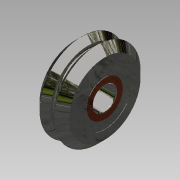
# Autodesk Inventor part: W3X
Saved by Autodesk Inventor 2020.1 (Build 241239000, 239)
## iProperties
Created: 2019-11-27
Part Number: W3X
Material: Generic
Catalog Web Link: https://www.bwc.com/dualvee.html
Vendor: BWC
Document SubType Name: Modeling
Designer: Autodesk Inc.
Manufacturer: BWC
Mass: 130.2 g
Surface Area: 59.8551 cm^2
Volume: 19.8505 cm^3
Density: 1 g/cm^3
Appearance: PSOLRGB-175-175-175
Category: FIRSTChoice
Company: Autodesk Inc.
PSOL_IDENT_0: {$CADENAS_DATA\23d-libs\bwc\dual_vee\wheels\original_dualvee_wheels.prj},163 {VTYP=3D},{NB=W3X},{LIN
PSOL_IDENT_1: A=W3X},{NN=Original DualVee Wheels},{DATE=01.07.2019 05:07:11},{GEOMDATE=12.02.2019 13:07:27},{VERSI
PSOL_IDENT_2: ON=},{LINEID=40},{WBVAR=},{WBNUMERIC=}  {NB=W3X},{LINA=W3X},{KT=DUMMY},{PN=W3X},{WS=WX Steel Seal/Sh
PSOL_IDENT_3: ield},{WSPN=X},{WSALG= 'X','WX Seal/Shield Steel', 'SSX','WSSX Seal/Shield Stainless Steel','SS227',
PSOL_IDENT_4: 'WSS227 Shield Stainless Steel Krytox GPL227 Lubricant','SS300', 'WSS300 Stainless Steel Isoflex PD
PSOL_IDENT_5: L 300 (grease, no shields or seals)','DW3SSX', 'Washdown Sealed Wheels' },{SIZE=3},{D=1.803},{W=0.62
PSOL_IDENT_6: 5},{B=0.4724},{VRI=0.750},{VRO=1.063},{WEIGHT=130.2},{C=0.755},{R=0.039},{R1=0.024},{E=0.010},{RLN=5
PSOL_IDENT_7: 900},{RLLBF=1326},{ALN=1701},{ALLBF=382},{ORMAT=52100 Steel},{IRMAT=52100 Steel},{BMAT=52100 Steel},
PSOL_IDENT_8: {RMAT=Nylon 6,6},{SHMAT=304 Stainless steel},{SMAT=NBR+304 Stainless steel},{GREASE=Kluberplex BEM 3
PSOL_IDENT_9: 4-132},{CFGFILTER=PN,WS,SIZE,D,W,B,VRI,VRO,WEIGHT,RLN,RLLBF,ALN,ALLBF,ORMAT,IRMAT,BMAT,RMAT,SHMAT,SM
PSOL_IDENT_10: AT,GREASE},{CATEGALG=Original Guide Wheel, Size 3, Carbon Steel, Sealed/Shielded},{FEATALG=<li style=
PSOL_IDENT_11: \" margin-top:0px; margin-bottom:0px; margin-left:0px; margin-right:0px; -qt-block-indent:0; text-in
PSOL_IDENT_12: dent:0px;\"><span style=\" font-size:11pt; font-weight:600;\">General purpose AISI 52100 carbon stee
PSOL_IDENT_13: l</span></li><li style=\" font-size:11pt; font-weight:600;\" style=\" margin-top:0px; margin-bottom:
PSOL_IDENT_14: 0px; margin-left:0px; margin-right:0px; -qt-block-indent:0; text-indent:0px;\">Double row angular co
PSOL_IDENT_15: ntact ball bearing</li><li style=\" font-size:11pt; font-weight:600;\" style=\" margin-top:0px; marg
PSOL_IDENT_16: in-bottom:0px; margin-left:0px; margin-right:0px; -qt-block-indent:0; text-indent:0px;\">Precision g
PSOL_IDENT_17: round 90° vee inside or outside running surfaces</li><li style=\" font-size:11pt; font-weight:600;\"
PSOL_IDENT_18: style=\" margin-top:0px; margin-bottom:0px; margin-left:0px; margin-right:0px; -qt-block-indent:0;
PSOL_IDENT_19: text-indent:0px;\">Hardened for heavy loads and durability</li><li style=\" font-size:11pt; font-wei
PSOL_IDENT_20: ght:600;\" style=\" margin-top:0px; margin-bottom:0px; margin-left:0px; margin-right:0px; -qt-block-
PSOL_IDENT_21: indent:0; text-indent:0px;\">Seal/Shield combination to protect against contamination</li>},{DESCRAL
PSOL_IDENT_22: G=<span style=\" font-size:11pt; font-weight:600;\">DualVee WX series guide wheels are linear guide
PSOL_IDENT_23: bearings with double row angular contact ball arrangement.   Precision ground 90° vee inside or outs
PSOL_IDENT_24: ide surfaces can be employed to support loads and provide smooth and quiet motion. Use with DualVee
PSOL_IDENT_25: guide track for linear motion. Hybrid seal/shield design with rubber inner seal and metal outer shie
PSOL_IDENT_26: ld protects against particle contamination of all sizes. Through bore allows mounting on bushings or
PSOL_IDENT_27: journals. Internally lubricated with general purpose grease.</span>},{RATINGSALG=<span style=\" fon
PSOL_IDENT_28: t-size:11pt; font-weight:600; color:#000000;\">Temperature Range:</span><span style=\" font-size:11p
PSOL_IDENT_29: t; color:#000000;\"> -22°F to +212°F</span></p><p style=\" margin-top:0px; margin-bottom:0px; margin
PSOL_IDENT_30: -left:0px; margin-right:0px; -qt-block-indent:0; text-indent:0px;\"><span style=\" font-size:11pt; f
PSOL_IDENT_31: ont-weight:600; color:#000000;\">RoHS Compliant</span>},{MATCOLALG=ORMAT( title=\"$var. ($desc.)\",
PSOL_IDENT_32: format=\"$value(SRC=VALDESC).\" ),IRMAT( title=\"$var. ($desc.)\", format=\"$value(SRC=VALDESC).\" )
PSOL_IDENT_33: ,BMAT( title=\"$var. ($desc.)\", format=\"$value(SRC=VALDESC).\" ),RMAT( title=\"$var. ($desc.)\", f
PSOL_IDENT_34: ormat=\"$value(SRC=VALDESC).\" ),SHMAT( title=\"$var. ($desc.)\", format=\"$value(SRC=VALDESC).\" ),
PSOL_IDENT_35: SMAT( title=\"$var. ($desc.)\", format=\"$value(SRC=VALDESC).\" ),GREASE( title=\"$var. ($desc.)\",
PSOL_IDENT_36: format=\"$value(SRC=VALDESC).\" )},{MATCOL1=ORMAT( title=\"$var. ($desc.)\", format=\"$value(SRC=VAL
PSOL_IDENT_37: DESC).\" ),IRMAT( title=\"$var. ($desc.)\", format=\"$value(SRC=VALDESC).\" ),BMAT( title=\"$var. ($
PSOL_IDENT_38: desc.)\", format=\"$value(SRC=VALDESC).\" ),RMAT( title=\"$var. ($desc.)\", format=\"$value(SRC=VALD
PSOL_IDENT_39: ESC).\" ),SHMAT( title=\"$var. ($desc.)\", format=\"$value(SRC=VALDESC).\" ),SMAT( title=\"$var. ($d
PSOL_IDENT_40: esc.)\", format=\"$value(SRC=VALDESC).\" ),GREASE( title=\"$var. ($desc.)\", format=\"$value(SRC=VAL
PSOL_IDENT_41: DESC).\" )}
NN: Original DualVee Wheels
NT: Original DualVee Wheels
NB: W3X
NBSYN: $PN.
LINA: W3X
PN: W3X
WS: WX Steel Seal/Shield
SIZE: 3
D: 1.803
W: 0.625
B: 0.4724
VRI: 0.75
VRO: 1.063
WEIGHT: 130.2
RLN: 5900
RLLBF: 1326
ALN: 1701
ALLBF: 382
ORMAT: 52100 Steel
IRMAT: 52100 Steel
BMAT: 52100 Steel
RMAT: Nylon 6,6
SHMAT: 304 Stainless steel
SMAT: NBR+304 Stainless steel
GREASE: Kluberplex BEM 34-132
SUPPLIER: BWC
ARTICLENO: W3X
BOMINFO: W3X
CREATOR: CADENAS GmbH
Author: Autodesk Inc.
Comments: Original DualVee Wheels
Autodesk Inventor part; units mm, degrees
sketch "Sketch_1" plane through (0, 0, 0) normal (0, 0, 1) x (1, 0, 0)
  line L0 (7.3279, 0) -> (-7.3279, 0)
  line L1 (-7.9375, 9.5885) -> (-7.9375, 6.6091)
  arc A0 (-7.9375, 6.6091) -> (-7.3279, 5.9995) centre (-7.3279, 6.6091) ccw
  line L2 (-7.3279, 5.9995) -> (7.3279, 5.9995)
  arc A1 (7.3279, 5.9995) -> (7.9375, 6.6091) centre (7.3279, 6.6091) ccw
  line L3 (7.9375, 6.6091) -> (7.9375, 9.5885)
  line L4 (7.9375, 9.5885) -> (7.8105, 9.5885)
  line L5 (7.8105, 9.5885) -> (7.8105, 9.4615)
  line L6 (7.8105, 9.4615) -> (7.6835, 9.4615)
  line L7 (7.6835, 9.4615) -> (7.6835, 14.4463)
  line L8 (7.6835, 14.4463) -> (7.8105, 14.4463)
  line L9 (7.8105, 14.4463) -> (7.8105, 14.3193)
  line L10 (7.8105, 14.3193) -> (7.9375, 14.3193)
  line L11 (7.9375, 14.3193) -> (7.9375, 19.05)
  line L12 (7.9375, 19.05) -> (4.0894, 22.8981)
  line L13 (4.0894, 22.8981) -> (3.8354, 22.8981)
  line L14 (3.8354, 22.8981) -> (0.9906, 20.0533)
  line L15 (0.9906, 20.0533) -> (0.9906, 19.05)
  arc A2 (-0.9906, 19.05) -> (0.9906, 19.05) centre (0, 19.05) ccw
  line L16 (-0.9906, 19.05) -> (-0.9906, 20.0533)
  line L17 (-0.9906, 20.0533) -> (-3.8354, 22.8981)
  line L18 (-3.8354, 22.8981) -> (-4.0894, 22.8981)
  line L19 (-4.0894, 22.8981) -> (-7.9375, 19.05)
  line L20 (-7.9375, 19.05) -> (-7.9375, 14.3193)
  line L21 (-7.9375, 14.3193) -> (-7.8105, 14.3193)
  line L22 (-7.8105, 14.3193) -> (-7.8105, 14.4463)
  line L23 (-7.8105, 14.4463) -> (-7.6835, 14.4463)
  line L24 (-7.6835, 14.4463) -> (-7.6835, 9.4615)
  line L25 (-7.6835, 9.4615) -> (-7.8105, 9.4615)
  line L26 (-7.8105, 9.4615) -> (-7.8105, 9.5885)
  line L27 (-7.8105, 9.5885) -> (-7.9375, 9.5885)
  constraints: 56 end point, 6 point on circle, 3 centre point
revolve "Revolution1" add sketch "Sketch_1" angle 360 about axis through (7.3279, 0, 0) along (1, 0, 0)
ref_plane "b_XY" through (-7.3279, 5.9995, 0) normal (0, 0, 1) x (1, 0, 0)
ref_plane "b_YZ" through (-7.3279, 5.9995, 0) normal (1, 0, 0) x (0, 1, 0)
ref_plane "b_ZX" through (-7.3279, 5.9995, 0) normal (0, 1, 0) x (0, 0, 1)
ref_plane "b1_XY" through (-7.3279, -5.9995, 0) normal (0, 0, 1) x (1, 0, 0)
ref_plane "b1_YZ" through (-7.3279, -5.9995, 0) normal (1, 0, 0) x (0, 1, 0)
ref_plane "b1_ZX" through (-7.3279, -5.9995, 0) normal (0, 1, 0) x (0, 0, 1)
ref_plane "d_XY" through (-3.9688, 22.8981, 0) normal (0, 0, 1) x (1, 0, 0)
ref_plane "d_YZ" through (-3.9688, 22.8981, 0) normal (1, 0, 0) x (0, 1, 0)
ref_plane "d_ZX" through (-3.9688, 22.8981, 0) normal (0, 1, 0) x (0, 0, 1)
ref_plane "d1_XY" through (-3.9688, -22.8981, 0) normal (0, 0, 1) x (1, 0, 0)
ref_plane "d1_YZ" through (-3.9688, -22.8981, 0) normal (1, 0, 0) x (0, 1, 0)
ref_plane "d1_ZX" through (-3.9688, -22.8981, 0) normal (0, 1, 0) x (0, 0, 1)
ref_plane "vri_XY" through (0, 19.05, 0) normal (0, 0, 1) x (1, 0, 0)
ref_plane "vri_YZ" through (0, 19.05, 0) normal (1, 0, 0) x (0, 1, 0)
ref_plane "vri_ZX" through (0, 19.05, 0) normal (0, 1, 0) x (0, 0, 1)
ref_plane "vri1_XY" through (7.9375, 0, 0) normal (0, 0, 1) x (1, 0, 0)
ref_plane "vri1_YZ" through (7.9375, 0, 0) normal (1, 0, 0) x (0, 1, 0)
ref_plane "vri1_ZX" through (7.9375, 0, 0) normal (0, 1, 0) x (0, 0, 1)
ref_plane "w_XY" through (-7.9375, 19.05, 0) normal (0, 0, 1) x (1, 0, 0)
ref_plane "w_YZ" through (-7.9375, 19.05, 0) normal (1, 0, 0) x (0, 1, 0)
ref_plane "w_ZX" through (-7.9375, 19.05, 0) normal (0, 1, 0) x (0, 0, 1)
ref_plane "w1_XY" through (7.9375, 19.05, 0) normal (0, 0, 1) x (1, 0, 0)
ref_plane "w1_YZ" through (7.9375, 19.05, 0) normal (1, 0, 0) x (0, 1, 0)
ref_plane "w1_ZX" through (7.9375, 19.05, 0) normal (0, 1, 0) x (0, 0, 1)
ref_plane "wheel_XY" through (7.9375, 0, 0) normal (1, 0, 0) x (0, 0, -1)
ref_plane "wheel_YZ" through (7.9375, 0, 0) normal (0, 0, -1) x (0, 1, 0)
ref_plane "wheel_ZX" through (7.9375, 0, 0) normal (0, 1, 0) x (1, 0, 0)
ref_plane "wheel2_XY" through (-7.9375, 0, 0) normal (1, 0, 0) x (0, 0, -1)
ref_plane "wheel2_YZ" through (-7.9375, 0, 0) normal (0, 0, -1) x (0, 1, 0)
ref_plane "wheel2_ZX" through (-7.9375, 0, 0) normal (0, 1, 0) x (1, 0, 0)
body "Solid1"
